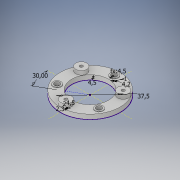
# Autodesk Inventor part: PlanetaryHolderBottom
Saved by Autodesk Inventor 2018.3 (Build 223284000, 284)
## iProperties
Created: 2018-07-08
Part Number: PlanetaryHolderBottom
Material: Generisch
Document SubType Name: Modeling
Designer: JochenAlt
Density: 1 g/cm^3
Appearance: Vorgabe
Author: JochenAlt
Autodesk Inventor part; units mm, degrees
ref_plane "YZ Plane" through (0, 0, 0) normal (1, 0, 0) x (0, 1, 0)
ref_plane "XZ Plane" through (0, 0, 0) normal (0, 1, 0) x (-1, 0, 0)
ref_plane "XY Plane" through (0, 0, 0) normal (0, 0, 1) x (1, 0, 0)
sketch "Skizze1" plane through (0, 0, 0) normal (0, 0, 1) x (1, 0, 0)
  line L0 (-32.55, 0) -> (32.55, 0) construction
  circle A0 centre (0, 0) radius 18.75 construction
  circle A1 centre (0, 18.75) radius 2.1
  circle A2 centre (16.238, -9.375) radius 2.1
  circle A3 centre (-16.238, -9.375) radius 2.1
  line L1 (0, 32.55) -> (0, -32.55) construction
  line L2 (0, 0) -> (-16.238, -9.375) construction
  circle A4 centre (0, 0) radius 14.25
  circle A5 centre (0, 0) radius 23.25
  circle A6 centre (0, -18.75) radius 1.15
  circle A7 centre (16.238, 9.375) radius 1.15
  circle A8 centre (-16.238, 9.375) radius 1.15
  circle A9 centre (0, -18.75) radius 4.25
  circle A10 centre (-16.238, 9.375) radius 4.25
  circle A11 centre (16.238, 9.375) radius 4.25
  circle A12 centre (0, -18.75) radius 2.25
  circle A13 centre (-16.238, 9.375) radius 2.25
  circle A14 centre (16.238, 9.375) radius 2.25
  circle A15 centre (16.238, -9.375) radius 3.1
  circle A16 centre (0, 18.75) radius 3.1
  circle A17 centre (-16.238, -9.375) radius 3.1
  dimension "d0" = 37.5
  dimension "d1" = 4.2
  dimension "d2" = 30
  dimension "d3" = 4.5
  dimension "d4" = 4.5
  dimension "d9" = 2.3
  dimension "d14" = 2
  dimension "d15" = 4.5
  dimension "d18" = 1
  constraints: 17 centre point, 11 coincident, 10 equal radius, 2 end point, 2 point on line, 1 symmetric about line, 10 other
  measures "d1" diameter of A1
  measures "d2" angle of L2 L0
  measures "d9" diameter of A6
  measures "d14" radial gap between concentric circles of A9 A12
  measures "d15" diameter of A12
  measures "d18" radial gap between concentric circles of A16 A1
extrude "Extrusion2" add sketch "Skizze1" along normal blind 1.5 contours A1 | A2 | A3 | A5 | A9 | A10 | A11 | A15 | A16 | A17
extrude "Extrusion1" add sketch "Skizze1" along normal blind 2 from surface at 1.5 contours A5 | A9 | A10 | A11 | A12 | A13 | A14 | A15 | A16 | A17
extrude "Extrusion3" add sketch "Skizze1" along normal blind 3 from surface at 3.5 contours A9 | A10 | A11 | A12 | A13 | A14
extrude "Extrusion4" add sketch "Skizze1" along normal blind 0.5 from surface at 3.5 contours A15 | A16 | A17
equation "\"d3\" = d4"
